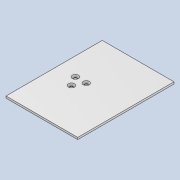
# Autodesk Inventor part: Board
Saved by Autodesk Inventor 2022 (Build 260153000, 153)
## iProperties
Created: 2023-06-19
Part Number: Board
Material: アルミニウム 2014-T4
Document SubType Name: Modeling
Designer: 81805
Density: 2.8 g/cm^3
Appearance: サテン
Author: 81805
Autodesk Inventor part; units mm, degrees
ref_plane "YZ Plane" through (0, 0, 0) normal (1, 0, 0) x (0, 1, 0)
ref_plane "XZ Plane" through (0, 0, 0) normal (0, 1, 0) x (-1, 0, 0)
ref_plane "XY Plane" through (0, 0, 0) normal (0, 0, 1) x (1, 0, 0)
sketch "スケッチ1" plane through (0, 0, 0) normal (0, 0, 1) x (1, 0, 0)
  line L0 (-100, 74.5) -> (100, 74.5)
  line L1 (100, 74.5) -> (100, -74.5)
  line L2 (100, -74.5) -> (-100, -74.5)
  line L3 (-100, -74.5) -> (-100, 74.5)
  line L4 (-100, 74.5) -> (100, -74.5) construction
  line L5 (100, 74.5) -> (-100, -74.5) construction
  circle A0 centre (0, -25.5) radius 13
  point P0 (0, 0)
  point P1 (13, -25.5)
  point P2 (-6.5, -14.2417)
  point P3 (-6.5, -36.7583)
  dimension "d4" = 26
  dimension "d0" = 200
  dimension "d1" = 149
  dimension "d10" = 360
  dimension "d19" = 100
  dimension "d20" = 49
  dimension "d22" = 0
  constraints: 12 end point, 2 midpoint, 2 parallel, 1 horizontal, 1 horizontal alignment, 1 perpendicular, 6 other
  measures "d0" distance of L0.start L0.end
  measures "d1" distance of L2.end L0.start
  measures "d19" distance from line of point (0, -25.5) L3
  measures "d20" distance from line of L2 point (0, -25.5)
  measures "d22" vertical distance of point (0, -25.5) point (13, -25.5)
extrude "押し出し1" add sketch "スケッチ1" against normal blind 4 contours L0 L1 L2 L3 | A0
hole "穴1" at (13, -25.5, 0) at (-6.5, -14.2417, 0) at (-6.5, -36.7583, 0) direction (0, 0, -1) diameter 5.9436 depth 10.65 tip angle 118 countersink diameter 12.6 countersink angle 90 thread size "1/16" designation "1/16 - 27 NPT" standard "NPT for PVC Pipe and Fitting"
